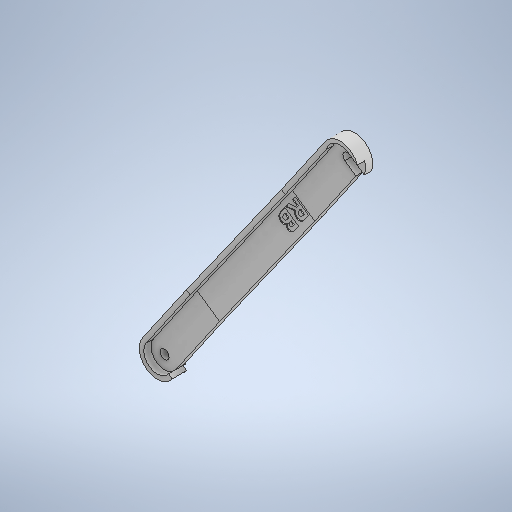
# Autodesk Inventor part: TheHandle_RightBack
Saved by Autodesk Inventor 2025.1 (Build 291241000, 241)
## iProperties
Created: 2026-05-10
Part Number: TheHandle_RightBack
Material: Generic
Document SubType Name: Modeling
Designer: User
Density: 1 g/cm^3
Appearance: Default
Author: User
## iProperties of the stored document TheHandle_RightBack_3DPrint.ipt
Created: 2026-05-12
Part Number: TheHandle_RightBack_3DPrint
Material: Generic
Document SubType Name: Modeling
Designer: User
Density: 1 g/cm^3
Appearance: Default
Author: User
Autodesk Inventor part; units mm, degrees
ref_plane "YZ Plane" through (0, 0, 0) normal (1, 0, 0) x (0, 1, 0)
ref_plane "XZ Plane" through (0, 0, 0) normal (0, 1, 0) x (-1, 0, 0)
ref_plane "XY Plane" through (0, 0, 0) normal (0, 0, 1) x (1, 0, 0)
sketch "Sketch1" plane through (0, 0, 0) normal (0, 0, 1) x (1, 0, 0)
  arc A0 (211.807006, -18.334947) -> (222.207006, -18.334947) centre (217.007006, -18.334947) ccw
  circle A1 centre (217.007006, -18.334947) radius 2.5
  circle A2 centre (120.003833, -158.855414) radius 2.5
  circle A3 centre (120.003833, -158.855414) radius 7.5
  circle A4 centre (217.007006, -18.334947) radius 7.5
  arc A5 (224.204489, -20.44356) -> (210.83481, -14.074197) centre (217.007006, -18.334947) ccw
  line L0 (126.176029, -163.116165) -> (223.179203, -22.595697)
  line L1 (210.83481, -14.074197) -> (113.831636, -154.594664)
  point P0 (0, 0)
  dimension "d0" = 5
  dimension "d1" = 15
  dimension "d2" = 15
  constraints: 4 end point, 4 point on circle, 4 tangent, 3 centre point, 3 coincident
  measures "d0" diameter of A1
  measures "d1" diameter of A3
  measures "d2" diameter of A4
extrude "Extrusion1" add sketch "Sketch1" along normal blind 4
sketch "Sketch2" plane through (223.179203, -22.595697, 4) normal (0.8229595, -0.5681, 0) x (0, 0, -1)
  line L0 (4, -170.750161) -> (4, 0)
  line L1 (4, 0) -> (0, 0)
  line L2 (0, -170.750161) -> (0, 0)
  line L3 (4, -170.750161) -> (0, -170.750161)
  line L4 (0, -85.375081) -> (4, -85.375081)
  line L5 (0, -170.750161) -> (0, 0)
  line L6 (0, -85.375081) -> (0, 0)
  line L7 (0, -42.68754) -> (4, -42.68754)
  line L8 (0, -170.750161) -> (0, -85.375081)
  line L9 (0, -128.062621) -> (4, -128.062621)
  line L10 (-4, -170.750161) -> (-4, 0)
  line L11 (4, -128.062621) -> (-4, -128.062621)
  line L12 (4, -85.375081) -> (-4, -85.375081)
  line L13 (0, -128.062621) -> (4, -42.68754)
  line L14 (0, -42.68754) -> (-4, -128.062621)
  line L15 (4, -170.750161) -> (-4, -170.750161)
  point P0 (4, -108.192771)
  point P1 (0, -170.750161)
  point P2 (0, -128.062621)
  dimension "d5" = 4
  constraints: 22 end point, 5 midpoint, 4 point on line, 3 perpendicular, 2 collinear, 1 parallel
  measures "d5" distance between parallel lines of L2 L10
extrude "Extrusion2" add sketch "Sketch2" against normal up to surface (15 mm away) contours L15 L10 L11 L2 | L11 L14 L12 L2 | L2 L4 L13 | L13 L4 L2 L7 | L12 L14 L2
sketch "Sketch3" plane through (223.179203, -22.595697, 4) normal (0.8229595, -0.5681, 0) x (0, 0, -1)
  line L0 (4, -170.750161) -> (0, -170.750161)
  line L1 (4, -170.750161) -> (4, 0)
  line L2 (4, 0) -> (0, 0)
  line L3 (0, -42.68754) -> (0, 0)
  line L4 (0, -42.68754) -> (-4, -128.062621)
  line L5 (-4, -128.062621) -> (-4, -170.750161)
  line L6 (-4, -170.750161) -> (0, -170.750161)
  line L7 (0, -170.750161) -> (0, -42.68754)
  line L8 (-4, -128.062621) -> (0, -128.062621)
  line L9 (-4, -128.062621) -> (0, -128.062621) construction
  line L10 (0, -42.68754) -> (4, -42.68754)
  line L11 (4, -42.68754) -> (0, -128.062621)
  line L12 (4, -178.250161) -> (4, -163.817796)
  line L13 (0, -166.489425) -> (0, -164.435585)
  line L14 (0, -178.250161) -> (4, -178.250161)
  point P0 (4, -108.192771)
  point P1 (1.449139, -170.750161)
  dimension "d8" = 0
  constraints: 10 end point, 2 collinear, 2 point on line, 1 horizontal, 1 perpendicular, 3 other
  measures "d8" distance between parallel lines of L8 L9
sketch "Sketch3 outline for Extrusion3" plane through (223.179203, -22.595697, 4) normal (0.8229595, -0.5681, 0) x (0, 0, -1)
  line L0 (0, -170.750161) -> (1.449139, -170.750161)
  line L1 (1.449139, -170.750161) -> (4, -178.250161)
  line L2 (4, -178.250161) -> (4, -42.68754)
  line L3 (4, -42.68754) -> (0, -128.062621)
  line L4 (0, -128.062621) -> (0, -170.750161)
extrude "Extrusion3" cut sketch "Sketch3 outline for Extrusion3" against normal through all
sketch "Sketch4" plane through (126.176029, -163.116165, 8) normal (0, 0, 1) x (0.8229595, -0.5681, 0)
  circle A0 centre (-7.5, 0) radius 2.5 projected
  point P0 (-196.504062, 62.55739)
extrude "Extrusion4" cut sketch "Sketch4" against normal blind 10
sketch "Sketch5" plane through (126.176029, -163.116165, 8) normal (0, 0, 1) x (0.8229595, -0.5681, 0)
  line L0 (0, 42.68754) -> (0, 0)
  line L1 (-15, 42.68754) -> (-15, 0)
  arc A0 (-5, 0) -> (-10, 0) centre (-7.5, 0) ccw
  circle A1 centre (-7.5, 0) radius 2.5
  circle A2 centre (-7.5, 0) radius 7.5
  point P0 (-196.504062, 62.55739)
  constraints: 1 coincident, 1 horizontal alignment, 2 other
extrude "Extrusion5" add sketch "Sketch5" against normal up to surface (4 mm away)
sketch "Sketch6" plane through (0, 0, 4) normal (0, 0, 1) x (1, 0, 0)
  circle A0 centre (217.007006, -18.334947) radius 2.5
  arc A1 (223.179203, -22.595697) -> (210.83481, -14.074197) centre (217.007006, -18.334947) ccw
  circle A2 centre (217.007006, -18.334947) radius 2.5
  line L0 (186.584017, -49.204314) -> (198.928409, -57.725814)
  line L1 (198.928409, -57.725814) -> (223.179203, -22.595697)
  arc A3 (223.179203, -22.595697) -> (210.83481, -14.074197) centre (217.007006, -18.334947) ccw
  line L2 (210.83481, -14.074197) -> (186.584017, -49.204314)
  circle A4 centre (120.003833, -158.855414) radius 2.5
  arc A5 (221.663941, -24.790732) -> (215.586756, -20.392346) centre (120.003833, -158.855414) ccw
  arc A6 (224.204489, -20.44356) -> (218.427256, -16.277548) centre (120.003833, -158.855414) ccw
  point P0 (0, 0)
  point P1 (224.204489, -20.44356)
  point P2 (218.427256, -16.277548)
  point P3 (215.586756, -20.392346)
  point P4 (223.179203, -22.595697)
  dimension "d15" = 5
  constraints: 7 point on circle, 2 centre point, 1 coincident, 1 point on line, 1 tangent
  measures "d15" radial gap between concentric circles of A5 A6
extrude "Extrusion6" cut sketch "Sketch6" against normal blind 10 contours A0 A6 A1 L1 A5
sketch "Sketch7" plane through (0, 0, 4) normal (0, 0, 1) x (1, 0, 0)
  arc A0 (224.204489, -20.44356) -> (210.83481, -14.074197) centre (217.007006, -18.334947) ccw
  line L0 (210.83481, -14.074197) -> (186.584017, -49.204314)
  arc A1 (224.204489, -20.44356) -> (218.427256, -16.277548) centre (120.003833, -158.855414) ccw
  line L1 (184.526618, -47.784063) -> (208.777411, -12.653947)
  arc A2 (225.066718, -24.254495) -> (208.777411, -12.653947) centre (217.007006, -18.334947) ccw
  arc A3 (225.066718, -24.254495) -> (217.007006, -18.334947) centre (120.003833, -158.855414) ccw
  arc A4 (218.427256, -16.277548) -> (215.586756, -20.392346) centre (217.007006, -18.334947) ccw
  line L2 (186.584017, -49.204314) -> (208.777411, -12.653947)
  line L3 (218.427256, -16.277548) -> (224.204489, -20.44356)
  arc A5 (224.204489, -20.44356) -> (218.427256, -16.277548) centre (120.003833, -158.855414) ccw
  line L4 (218.427256, -16.277548) -> (226.322567, -21.970924)
  line L5 (184.526618, -47.784063) -> (186.584017, -49.204314)
  point P0 (0, 0)
  point P1 (224.204489, -20.44356)
  dimension "d18" = 2.5
  constraints: 10 end point, 5 point on circle, 2 centre point, 1 point on line, 2 other
  measures "d18" radial gap between concentric circles of A0 A2
extrude "Extrusion7" add sketch "Sketch7" along normal mid plane 8 contours A0 L0 L2 A2 L4 | L5 L1 L2
sketch "Sketch8" plane through (113.831636, -154.594664, 4) normal (-0.8229595, 0.5681, 0) x (0, 0, 1)
  line L0 (4, 0) -> (0, 0)
  line L1 (4, 0) -> (0, 0)
  line L2 (0, 128.062621) -> (4, 42.68754)
  line L3 (3.995617, 128.249824) -> (7.995617, 42.874743)
  line L4 (4, 42.68754) -> (4, 0)
  line L5 (8, 0) -> (8, 42.781193)
  line L6 (8, 42.781193) -> (3.995617, 128.249824)
  line L7 (-4, 128.062621) -> (0, 42.68754)
  line L8 (0, 42.68754) -> (0, 0)
  line L9 (8, 0) -> (0, 0)
  line L10 (0, 128.062621) -> (-4, 128.062621)
  line L11 (0, 128.062621) -> (4, 128.062621)
  line L12 (4, 128.062621) -> (4, 170.750161)
  line L13 (4, 128.062621) -> (-4, 128.062621)
  point P0 (-4, 62.55739)
  point P1 (7.995617, 42.874743)
  point P2 (4, 128.156274)
  point P3 (4, 0)
  dimension "d21" = 4
  dimension "d22" = 4
  constraints: 12 end point, 1 collinear, 1 horizontal, 1 parallel, 1 perpendicular, 1 other
  measures "d21" distance between parallel lines of L2 L3
  measures "d22" distance between parallel lines of L4 L5
extrude "Extrusion8" add sketch "Sketch8" along normal up to surface (2.5 mm away)
sketch "Sketch9" plane through (126.176029, -163.116165, 4) normal (0, 0, -1) x (-0.8229595, 0.5681, 0)
  arc A0 (0, 0) -> (15, 0) centre (7.5, 0) ccw projected
  arc A1 (-2.5, 0) -> (17.5, 0) centre (7.5, 0) ccw
  line L0 (-2.5, 0) -> (0, 0)
  line L1 (15, 0) -> (17.5, 0)
  point P0 (196.504062, 62.55739)
  dimension "d25" = 2.5
  constraints: 4 end point, 2 point on circle, 1 centre point, 1 collinear, 1 horizontal
  measures "d25" radial gap between concentric circles of A0 A1
extrude "Extrusion9" add sketch "Sketch9" against normal up to surface (8 mm away)
sketch "Sketch10" plane through (0, 0, 8) normal (0, 0, 1) x (1, 0, 0)
  arc A0 (224.204489, -20.44356) -> (210.83481, -14.074197) centre (217.007006, -18.334947) ccw
  line L0 (186.637221, -49.127241) -> (210.83481, -14.074197)
  arc A1 (224.684321, -20.584134) -> (210.42333, -13.790147) centre (217.007006, -18.334947) ccw
  line L1 (210.42333, -13.790147) -> (186.225741, -48.843191)
  circle A2 centre (217.007006, -18.334947) radius 8
  line L2 (198.928409, -57.725814) -> (221.663941, -24.790732)
  line L3 (217.007006, -18.334947) -> (225.606609, -5.877415)
  line L4 (221.551807, -11.751271) -> (229.733712, -17.39935)
  arc A3 (226.322567, -21.970924) -> (208.777411, -12.653947) centre (217.007006, -18.334947) ccw
  line L5 (224.204489, -20.44356) -> (226.322567, -21.970924)
  point P0 (0, 0)
  point P1 (226.489564, -15.159871)
  point P2 (221.551807, -11.751271)
  point P3 (210.42333, -13.790147)
  point P4 (209.253286, -16.365219)
  dimension "d28" = 0.5
  constraints: 6 end point, 2 point on circle, 1 centre point, 1 coincident, 1 parallel, 1 perpendicular, 1 point on line, 1 tangent, 6 other
  measures "d28" radial gap between concentric circles of A0 A1
extrude "Extrusion10" cut sketch "Sketch10" against normal up to surface (4 mm away) contours A0 L3 A1 A2 L5 | A0 L0 A2 A1 L3 | A2 A1 L4 A3 L5
sketch "Sketch11" plane through (150.426822, -127.986048, 8) normal (0.0265875, 0.0385151, 0.9989042) x (0.8229595, -0.5681, 0)
  line L0 (-3.385032, 85.444796) -> (-3.385032, 67.714202) construction
  line L1 (-3.385032, 67.714202) -> (-12.516732, 67.714202) construction
  line L2 (-12.516732, 67.714202) -> (-12.516732, 85.444796) construction
  line L3 (-12.516732, 85.444796) -> (-3.385032, 85.444796) construction
  line L4 (-12.516732, 76.061493) -> (-12.516732, 78.851324)
  line L5 (-12.516732, 78.851324) -> (-9.164495, 81.389551)
  line L6 (-9.164495, 81.389551) -> (-9.164495, 82.21836)
  line L7 (-9.164495, 82.21836) -> (-12.516732, 82.21836)
  line L8 (-12.516732, 82.21836) -> (-12.516732, 84.497585)
  line L9 (-12.516732, 84.497585) -> (-3.385032, 84.497585)
  line L10 (-3.385032, 84.497585) -> (-3.385032, 80.827145)
  spline S0 degree 2 poles (-3.385032, 80.827145) (-3.385032, 80.064937) (-3.577434, 78.940125) (-3.873437, 78.459119) knots 0 0 0 1 2 2 2
  spline S1 degree 2 poles (-3.873437, 78.459119) (-4.184241, 77.970714) (-5.153651, 77.393508) (-5.89366, 77.393508) knots 0 0 0 1 2 2 2
  spline S2 degree 2 poles (-5.89366, 77.393508) (-6.937071, 77.393508) (-8.246885, 78.340718) (-8.631689, 79.132527) knots 0 0 0 1 2 2 2
  line L11 (-8.631689, 79.132527) -> (-12.516732, 76.061493)
  spline S3 degree 2 poles (-6.182263, 79.746733) (-5.834459, 79.746733) (-5.338654, 80.013136) (-5.205452, 80.31654) knots 0 0 0 1 2 2 2
  spline S4 degree 2 poles (-5.205452, 80.31654) (-5.116651, 80.531142) (-5.064851, 81.056548) (-5.064851, 81.448752) knots 0 0 0 1 2 2 2
  line L12 (-5.064851, 81.448752) -> (-5.064851, 82.21836)
  line L13 (-5.064851, 82.21836) -> (-7.521677, 82.21836)
  line L14 (-7.521677, 82.21836) -> (-7.521677, 81.559753)
  spline S5 degree 2 poles (-7.521677, 81.559753) (-7.521677, 81.086148) (-7.403276, 80.412741) (-7.218274, 80.183338) knots 0 0 0 1 2 2 2
  spline S6 degree 2 poles (-7.218274, 80.183338) (-7.040672, 79.961336) (-6.567067, 79.746733) (-6.182263, 79.746733) knots 0 0 0 1 2 2 2
  spline S7 degree 2 poles (-9.719501, 68.084206) (-10.400309, 68.084206) (-11.42892, 68.602212) (-11.769324, 69.031416) knots 0 0 0 1 2 2 2
  spline S8 degree 2 poles (-11.769324, 69.031416) (-12.176328, 69.549422) (-12.516732, 70.777835) (-12.516732, 71.732446) knots 0 0 0 1 2 2 2
  line L15 (-12.516732, 71.732446) -> (-12.516732, 75.380686)
  line L16 (-12.516732, 75.380686) -> (-3.385032, 75.380686)
  line L17 (-3.385032, 75.380686) -> (-3.385032, 72.161651)
  spline S9 degree 2 poles (-3.385032, 72.161651) (-3.385032, 71.15524) (-3.540434, 70.119228) (-3.784637, 69.667823) knots 0 0 0 1 2 2 2
  spline S10 degree 2 poles (-3.784637, 69.667823) (-4.043639, 69.172018) (-4.931649, 68.691013) (-5.508855, 68.691013) knots 0 0 0 1 2 2 2
  spline S11 degree 2 poles (-5.508855, 68.691013) (-6.174863, 68.691013) (-7.218274, 69.35702) (-7.462477, 69.949026) knots 0 0 0 1 2 2 2
  line L18 (-7.462477, 69.949026) -> (-7.506877, 69.949026)
  spline S12 degree 2 poles (-7.506877, 69.949026) (-7.684479, 69.098017) (-8.787091, 68.084206) (-9.719501, 68.084206) knots 0 0 0 1 2 2 2
  spline S13 degree 2 poles (-9.682501, 70.452232) (-9.253296, 70.452232) (-8.772291, 70.792636) (-8.64649, 71.133039) knots 0 0 0 1 2 2 2
  spline S14 degree 2 poles (-8.64649, 71.133039) (-8.565089, 71.340242) (-8.550289, 72.07285) (-8.550289, 72.679656) knots 0 0 0 1 2 2 2
  line L19 (-8.550289, 72.679656) -> (-8.550289, 73.101461)
  line L20 (-8.550289, 73.101461) -> (-10.851714, 73.101461)
  line L21 (-10.851714, 73.101461) -> (-10.851714, 72.975659)
  spline S15 degree 2 poles (-10.851714, 72.975659) (-10.851714, 72.08765) (-10.829514, 71.406842) (-10.674112, 71.051638) knots 0 0 0 1 2 2 2
  spline S16 degree 2 poles (-10.674112, 71.051638) (-10.53351, 70.740835) (-10.015505, 70.452232) (-9.682501, 70.452232) knots 0 0 0 1 2 2 2
  spline S17 degree 2 poles (-5.96026, 71.022038) (-5.738258, 71.022038) (-5.272053, 71.251441) (-5.168452, 71.488243) knots 0 0 0 1 2 2 2
  spline S18 degree 2 poles (-5.168452, 71.488243) (-5.064851, 71.710246) (-5.05005, 72.331852) (-5.05005, 72.946059) knots 0 0 0 1 2 2 2
  line L22 (-5.05005, 72.946059) -> (-5.05005, 73.101461)
  line L23 (-5.05005, 73.101461) -> (-6.988872, 73.101461)
  line L24 (-6.988872, 73.101461) -> (-6.988872, 72.812858)
  spline S19 degree 2 poles (-6.988872, 72.812858) (-6.988872, 72.228251) (-6.966671, 71.754646) (-6.84827, 71.503043) knots 0 0 0 1 2 2 2
  spline S20 degree 2 poles (-6.84827, 71.503043) (-6.715069, 71.22924) (-6.263664, 71.022038) (-5.96026, 71.022038) knots 0 0 0 1 2 2 2
  point P0 (-196.504062, 20.222484)
  constraints: 2 other
emboss "Emboss1" sketch "Sketch11" operation cut depth 0.5 direction (-0.0265875, -0.0385151, -0.9989042)
body "Solid1"
